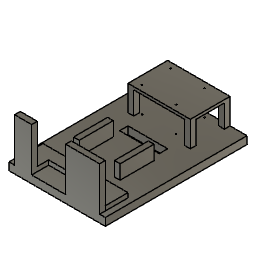
Partie_Haute_imprimable.f3d v1 (Autodesk Fusion 360 design; units mm, degrees)
Autodesk Fusion 360 part; units mm, degrees
form "Forme1" [no effect]
sketch "Sketch14" plane through (0, 0, 123.5) normal (0, 0, 1) x (-1, 0, 0)
  line L0 (-85, 80) -> (-85, -75)
  line L1 (80, -100) -> (-90, -100)
  line L2 (-90, -100) -> (-90, 150)
  line L3 (-90, 150) -> (80, 150)
  line L4 (80, 150) -> (80, -100)
  line L5 (-85, -75) -> (-70, -75)
  line L6 (-70, 80) -> (-85, 80)
  line L7 (-70, -75) -> (-70, 80)
  constraint horizontal L1
  constraint vertical L2
  constraint horizontal L3
  constraint vertical L4
extrude "Extrude16" add sketch "Sketch14" along normal blind 10 contours L0 L5 L6 L7 | L1 L2 L3 L4
sketch "Esquisse43" plane through (0, 0, 133.5) normal (0, 0, 1) x (-1, 0, 0)
  line L0 (80, -100) -> (80, 150)
  line L1 (-90, 150) -> (-90, -100)
  line L2 (-90, -100) -> (80, -100)
  line L3 (50, -100) -> (40, -100)
  line L4 (40, -100) -> (40, -90)
  line L5 (40, -90) -> (50, -90)
  line L6 (50, -90) -> (50, -100)
  line L7 (-60, -100) -> (-50, -100)
  line L8 (-50, -100) -> (-50, -90)
  line L9 (-50, -90) -> (-60, -90)
  line L10 (-60, -90) -> (-60, -100)
  line L11 (50, -40) -> (40, -40)
  line L12 (40, -40) -> (40, -30)
  line L13 (40, -30) -> (50, -30)
  line L14 (50, -30) -> (50, -40)
  line L15 (-60, -40) -> (-50, -40)
  line L16 (-50, -40) -> (-50, -30)
  line L17 (-50, -30) -> (-60, -30)
  line L18 (-60, -30) -> (-60, -40)
  line L19 (80, 150) -> (-90, 150)
  constraint horizontal L3
  constraint vertical L4
  constraint horizontal L5
  constraint vertical L6
  constraint horizontal L7
  constraint vertical L8
  constraint horizontal L9
  constraint vertical L10
  constraint horizontal L11
  constraint vertical L12
  constraint horizontal L13
  constraint vertical L14
  constraint horizontal L15
  constraint vertical L16
  constraint horizontal L17
  constraint vertical L18
extrude "Extrusion42" add sketch "Esquisse43" along normal blind 40 contours L2 L3 L4 L5 L6 | L2 L7 L8 L9 L10 | L11 L12 L13 L14 | L15 L16 L17 L18
sketch "Esquisse44" plane through (0, 0, 173.5) normal (0, 0, 1) x (-1, 0, 0)
  line L0 (50, -90) -> (40, -90)
  line L1 (40, -90) -> (40, -100)
  line L2 (40, -100) -> (50, -100)
  line L3 (50, -100) -> (50, -90)
  line L4 (50, -100) -> (-60, -100)
  line L5 (-60, -100) -> (-60, -30)
  line L6 (-60, -30) -> (50, -30)
  line L7 (50, -30) -> (50, -100)
  constraint horizontal L4
  constraint vertical L5
  constraint horizontal L6
  constraint vertical L7
  constraint coincident L2.end L3.start
extrude "Extrusion43" add sketch "Esquisse44" along normal blind 5
sketch "Esquisse45" plane through (0, 0, 133.5) normal (0, 0, 1) x (-1, 0, 0)
  line L0 (50, -30) -> (50, -40)
  line L1 (50, -40) -> (40, -40)
  line L2 (40, -40) -> (40, -30)
  line L3 (40, -30) -> (50, -30)
  line L4 (40, -100) -> (40, -90)
  line L5 (40, -90) -> (50, -90)
  line L6 (50, -90) -> (50, -100)
  line L7 (50, -100) -> (80, -100)
  line L8 (80, -100) -> (80, 150)
  line L9 (-90, 150) -> (-90, -100)
  line L10 (-90, -100) -> (-60, -100)
  line L11 (-60, -100) -> (-60, -90)
  line L12 (-60, -90) -> (-50, -90)
  line L13 (-50, -90) -> (-50, -100)
  line L14 (-50, -100) -> (40, -100)
  line L15 (-60, -30) -> (-50, -30)
  line L16 (-50, -30) -> (-50, -40)
  line L17 (-50, -40) -> (-60, -40)
  line L18 (-60, -40) -> (-60, -30)
  line L19 (30, -10) -> (-40, -10)
  line L20 (-40, -10) -> (-40, 4.8051)
  line L21 (-40, 4.8051) -> (30, 4.8051)
  line L22 (30, 4.8051) -> (30, -10)
  line L23 (80, 150) -> (-90, 150)
  constraint horizontal L19
  constraint vertical L20
  constraint horizontal L21
  constraint vertical L22
extrude "Extrusion44" cut sketch "Esquisse45" against normal blind 15 contours L19 L20 L21 L22
sketch "Esquisse47" plane through (0, 0, 133.5) normal (0, 0, 1) x (-1, 0, 0)
  line L0 (-40, -10) -> (-40, 4.8051)
  line L1 (-40, 4.8051) -> (30, 4.8051)
  line L2 (30, 4.8051) -> (30, -10)
  line L3 (30, -10) -> (-40, -10)
  line L4 (50, -30) -> (50, -40)
  line L5 (50, -40) -> (40, -40)
  line L6 (40, -40) -> (40, -30)
  line L7 (40, -30) -> (50, -30)
  line L8 (40, -100) -> (40, -90)
  line L9 (40, -90) -> (50, -90)
  line L10 (50, -90) -> (50, -100)
  line L11 (50, -100) -> (80, -100)
  line L12 (80, -100) -> (80, 150)
  line L13 (-90, 150) -> (-90, -100)
  line L14 (-90, -100) -> (-60, -100)
  line L15 (-60, -100) -> (-60, -90)
  line L16 (-60, -90) -> (-50, -90)
  line L17 (-50, -90) -> (-50, -100)
  line L18 (-50, -100) -> (40, -100)
  line L19 (-60, -30) -> (-50, -30)
  line L20 (-50, -30) -> (-50, -40)
  line L21 (-50, -40) -> (-60, -40)
  line L22 (-60, -40) -> (-60, -30)
  line L23 (36, 20) -> (26, 20)
  line L24 (26, 20) -> (26, 80)
  line L25 (26, 80) -> (36, 80)
  line L26 (36, 80) -> (36, 20)
  line L27 (-46, 20) -> (-36, 20)
  line L28 (-36, 20) -> (-36, 80)
  line L29 (-36, 80) -> (-46, 80)
  line L30 (-46, 80) -> (-46, 20)
  line L31 (80, 150) -> (-90, 150)
  constraint horizontal L23
  constraint vertical L24
  constraint horizontal L25
  constraint vertical L26
  constraint horizontal L27
  constraint vertical L28
  constraint horizontal L29
  constraint vertical L30
extrude "Extrusion46" add sketch "Esquisse47" along normal blind 25 contours L23 L24 L25 L26 | L27 L28 L29 L30
sketch "Esquisse48" plane through (0, 0, 133.5) normal (0, 0, 1) x (-1, 0, 0)
  line L0 (-46, 80) -> (-36, 80)
  line L1 (-36, 80) -> (-36, 20)
  line L2 (-36, 20) -> (-46, 20)
  line L3 (-46, 20) -> (-46, 80)
  line L4 (36, 80) -> (36, 20)
  line L5 (36, 20) -> (26, 20)
  line L6 (26, 20) -> (26, 80)
  line L7 (26, 80) -> (36, 80)
  line L8 (-40, -10) -> (-40, 4.8051)
  line L9 (-40, 4.8051) -> (30, 4.8051)
  line L10 (30, 4.8051) -> (30, -10)
  line L11 (30, -10) -> (-40, -10)
  line L12 (50, -30) -> (50, -40)
  line L13 (50, -40) -> (40, -40)
  line L14 (40, -40) -> (40, -30)
  line L15 (40, -30) -> (50, -30)
  line L16 (40, -100) -> (40, -90)
  line L17 (40, -90) -> (50, -90)
  line L18 (50, -90) -> (50, -100)
  line L19 (50, -100) -> (80, -100)
  line L20 (80, -100) -> (80, 150)
  line L21 (-90, 150) -> (-90, -100)
  line L22 (-90, -100) -> (-60, -100)
  line L23 (-60, -100) -> (-60, -90)
  line L24 (-60, -90) -> (-50, -90)
  line L25 (-50, -90) -> (-50, -100)
  line L26 (-50, -100) -> (40, -100)
  line L27 (-60, -30) -> (-50, -30)
  line L28 (-50, -30) -> (-50, -40)
  line L29 (-50, -40) -> (-60, -40)
  line L30 (-60, -40) -> (-60, -30)
  line L31 (70, 100) -> (-80, 100)
  line L32 (-80, 100) -> (-80, 140)
  line L33 (-80, 140) -> (70, 140)
  line L34 (70, 140) -> (70, 100)
  line L35 (80, 150) -> (-90, 150)
  constraint horizontal L31
  constraint vertical L32
  constraint horizontal L33
  constraint vertical L34
extrude "Extrusion47" add sketch "Esquisse48" along normal blind 8 contours L31 L32 L33 L34
sketch "Esquisse49" plane through (0, 0, 141.5) normal (0, 0, 1) x (-1, 0, 0)
  line L0 (70, 140) -> (-80, 140)
  line L1 (-80, 140) -> (-80, 100)
  line L2 (-80, 100) -> (70, 100)
  line L3 (70, 100) -> (70, 140)
  line L4 (40, 120) -> (-20, 120)
  line L5 (-20, 120) -> (-20, 140)
  line L6 (-20, 140) -> (40, 140)
  line L7 (40, 140) -> (40, 120)
  constraint horizontal L4
  constraint vertical L5
  constraint horizontal L6
  constraint vertical L7
extrude "Extrusion48" cut sketch "Esquisse49" against normal blind 8 contours L0 L4 L5 L6 L7
sketch "Esquisse50" plane through (0, 0, 133.5) normal (0, 0, 1) x (-1, 0, 0)
  line L0 (70, 140) -> (70, 100)
  line L1 (70, 100) -> (-80, 100)
  line L2 (-80, 100) -> (-80, 140)
  line L3 (-80, 140) -> (-20, 140)
  line L4 (-46, 80) -> (-36, 80)
  line L5 (-36, 80) -> (-36, 20)
  line L6 (-36, 20) -> (-46, 20)
  line L7 (-46, 20) -> (-46, 80)
  line L8 (36, 80) -> (36, 20)
  line L9 (36, 20) -> (26, 20)
  line L10 (26, 20) -> (26, 80)
  line L11 (26, 80) -> (36, 80)
  line L12 (-40, -10) -> (-40, 4.8051)
  line L13 (-40, 4.8051) -> (30, 4.8051)
  line L14 (30, 4.8051) -> (30, -10)
  line L15 (30, -10) -> (-40, -10)
  line L16 (50, -30) -> (50, -40)
  line L17 (50, -40) -> (40, -40)
  line L18 (40, -40) -> (40, -30)
  line L19 (40, -30) -> (50, -30)
  line L20 (40, -100) -> (40, -90)
  line L21 (40, -90) -> (50, -90)
  line L22 (50, -90) -> (50, -100)
  line L23 (50, -100) -> (80, -100)
  line L24 (80, -100) -> (80, 150)
  line L25 (-90, 150) -> (-90, -100)
  line L26 (-90, -100) -> (-60, -100)
  line L27 (-60, -100) -> (-60, -90)
  line L28 (-60, -90) -> (-50, -90)
  line L29 (-50, -90) -> (-50, -100)
  line L30 (-50, -100) -> (40, -100)
  line L31 (-60, -30) -> (-50, -30)
  line L32 (-50, -30) -> (-50, -40)
  line L33 (-50, -40) -> (-60, -40)
  line L34 (-60, -40) -> (-60, -30)
  line L35 (70, 140) -> (40, 140)
  line L36 (40, 140) -> (40, 150)
  line L37 (40, 150) -> (70, 150)
  line L38 (70, 150) -> (70, 140)
  line L39 (-20, 140) -> (-79.9271, 140)
  line L40 (-79.9271, 140) -> (-79.9271, 150)
  line L41 (-79.9271, 150) -> (-20, 150)
  line L42 (-20, 150) -> (-20, 140)
  line L43 (-20, 140) -> (-20, 120)
  line L44 (-20, 120) -> (40, 120)
  line L45 (40, 120) -> (40, 140)
  line L46 (40, 140) -> (70, 140)
  line L47 (80, 150) -> (-90, 150)
  constraint horizontal L35
  constraint vertical L36
  constraint horizontal L37
  constraint vertical L38
  constraint coincident L0.start L35.start
  constraint horizontal L39
  constraint vertical L40
  constraint horizontal L41
  constraint vertical L42
  constraint coincident L3.end L39.start
extrude "Extrusion49" add sketch "Esquisse50" along normal blind 77 contours L35 L36 L37 L38 L46 L47 | L3 L39 L40 L41 L42 L47
sketch "Esquisse54" plane through (0, 0, 178.5) normal (0, 0, 1) x (-1, 0, 0)
  line L0 (50, -30) -> (-60, -30)
  line L1 (-60, -30) -> (-60, -100)
  line L2 (-60, -100) -> (50, -100)
  line L3 (50, -100) -> (50, -30)
  circle A0 centre (35, -90) radius 1.25
  circle A1 centre (35, -40) radius 1.25
  circle A2 centre (-25, -90) radius 1.25
  circle A3 centre (-25, -40) radius 1.25
  dimension "d147" = 2.5
  dimension "d148" = 2.5
  dimension "d149" = 2.5
  dimension "d150" = 2.5
  measures "d147" diameter of A0
  measures "d148" diameter of A1
  measures "d149" diameter of A2
  measures "d150" diameter of A3
extrude "Extrusion52" cut sketch "Esquisse54" against normal blind 6 contours A0 | A1 | A2 | A3
sketch "Esquisse55" plane through (0, 0, 133.5) normal (0, 0, 1) x (-1, 0, 0)
  line L0 (-79.9271, 150) -> (-90, 150)
  line L1 (70, 150) -> (70, 100)
  line L2 (70, 100) -> (-80, 100)
  line L3 (-79.9271, 140) -> (-79.9271, 150)
  line L4 (-46, 80) -> (-36, 80)
  line L5 (-36, 80) -> (-36, 20)
  line L6 (-36, 20) -> (-46, 20)
  line L7 (-46, 20) -> (-46, 80)
  line L8 (36, 80) -> (36, 20)
  line L9 (36, 20) -> (26, 20)
  line L10 (26, 20) -> (26, 80)
  line L11 (26, 80) -> (36, 80)
  line L12 (-40, -10) -> (-40, 4.8051)
  line L13 (-40, 4.8051) -> (30, 4.8051)
  line L14 (30, 4.8051) -> (30, -10)
  line L15 (30, -10) -> (-40, -10)
  line L16 (50, -30) -> (50, -40)
  line L17 (50, -40) -> (40, -40)
  line L18 (40, -40) -> (40, -30)
  line L19 (40, -30) -> (50, -30)
  line L20 (40, -100) -> (40, -90)
  line L21 (40, -90) -> (50, -90)
  line L22 (50, -90) -> (50, -100)
  line L23 (50, -100) -> (80, -100)
  line L24 (80, -100) -> (80, 150)
  line L25 (-90, 150) -> (-90, -100)
  line L26 (-90, -100) -> (-60, -100)
  line L27 (-60, -100) -> (-60, -90)
  line L28 (-60, -90) -> (-50, -90)
  line L29 (-50, -90) -> (-50, -100)
  line L30 (-50, -100) -> (40, -100)
  line L31 (-60, -30) -> (-50, -30)
  line L32 (-50, -30) -> (-50, -40)
  line L33 (-50, -40) -> (-60, -40)
  line L34 (-60, -40) -> (-60, -30)
  circle A0 centre (35, -90) radius 1.25
  circle A1 centre (35, -40) radius 1.25
  circle A2 centre (-25, -90) radius 1.25
  circle A3 centre (-25, -40) radius 1.25
  line L35 (-80, 100) -> (-80, 140)
  line L36 (-80, 140) -> (-79.9271, 140)
  line L37 (80, 150) -> (70, 150)
  dimension "d153" = 2.5
  dimension "d154" = 2.5
  dimension "d155" = 2.5
  dimension "d156" = 2.5
  measures "d153" diameter of A0
  measures "d154" diameter of A1
  measures "d155" diameter of A2
  measures "d156" diameter of A3
extrude "Extrusion53" cut sketch "Esquisse55" against normal blind 15 contours A0 | A1 | A2 | A3
extrude "Extrusion54" add 1 faces at (16.6667, -101.6017, 123.5) along direction (0, 0, -1) blind 3.5
sketch "Esquisse56" plane through (0, 0, 120) normal (0, 0, -1) x (1, 0, 0)
  line L0 (40, 4.8051) -> (40, -10)
  line L1 (40, -10) -> (-30, -10)
  line L2 (-30, -10) -> (-30, 4.8051)
  line L3 (-30, 4.8051) -> (40, 4.8051)
  circle A0 centre (25, -40) radius 1.25
  circle A1 centre (-35, -40) radius 1.25
  line L4 (90, 150) -> (-80, 150)
  line L5 (-80, 150) -> (-80, -100)
  line L6 (-80, -100) -> (90, -100)
  line L7 (90, -100) -> (90, 150)
  circle A2 centre (25, -90) radius 1.25
  circle A3 centre (-35, -90) radius 1.25
  line L8 (-75, 145) -> (-60, 145)
  line L9 (-60, 145) -> (-60, 130)
  line L10 (-60, 130) -> (-75, 130)
  line L11 (-75, 130) -> (-75, 145)
  line L12 (70, 145) -> (85, 145)
  line L13 (85, 145) -> (85, 130)
  line L14 (85, 130) -> (70, 130)
  line L15 (70, 130) -> (70, 145)
  line L16 (-75, -75) -> (-60, -75)
  line L17 (-60, -75) -> (-60, -90)
  line L18 (-60, -90) -> (-75, -90)
  line L19 (-75, -90) -> (-75, -75)
  line L20 (70, -75) -> (85, -75)
  line L21 (85, -75) -> (85, -90)
  line L22 (85, -90) -> (70, -90)
  line L23 (70, -90) -> (70, -75)
  constraint horizontal L8
  constraint vertical L9
  constraint horizontal L10
  constraint vertical L11
  constraint horizontal L12
  constraint vertical L13
  constraint horizontal L14
  constraint vertical L15
  constraint horizontal L16
  constraint vertical L17
  constraint horizontal L18
  constraint vertical L19
  constraint horizontal L20
  constraint vertical L21
  constraint horizontal L22
  constraint vertical L23
extrude "Extrusion55" cut sketch "Esquisse56" against normal blind 5 contours L8 L9 L10 L11 | L12 L13 L14 L15 | L16 L17 L18 L19 | L20 L21 L22 L23
